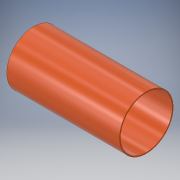
# Autodesk Inventor part: casting_tube
Saved by Autodesk Inventor 2017 SP1 (Build 210196100, 196)
## iProperties
Created: 2016-10-29
Part Number: casting_tube
Material: Phenolic Resin
Document SubType Name: Modeling
Designer: cflannery
Density: 1.38 g/cm^3
Appearance: Smooth - Light Orange
Author: cflannery
Autodesk Inventor part; units mm, degrees
ref_plane "YZ Plane" through (0, 0, 0) normal (1, 0, 0) x (0, 1, 0)
ref_plane "XZ Plane" through (0, 0, 0) normal (0, 1, 0) x (-1, 0, 0)
ref_plane "XY Plane" through (0, 0, 0) normal (0, 0, 1) x (1, 0, 0)
sketch "Sketch1" plane through (0, 0, 0) normal (1, 0, 0) x (0, 1, 0)
  circle A0 centre (0, 0) radius 90.805
  circle A1 centre (0, 0) radius 87.63
  dimension "d0" = 181.61
  dimension "d1" = 175.26
  constraints: 2 centre point, 2 coincident
  measures "d0" diameter of A0
  measures "d1" diameter of A1
extrude "Extrusion1" add sketch "Sketch1" along normal blind 381
body "Solid1"
